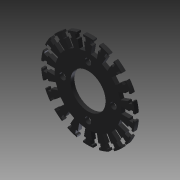
# Autodesk Inventor part: Plate 1
Saved by Autodesk Inventor 2015 (Build 190159000, 159)
## iProperties
Created: 2016-10-18
Part Number: Plate 1
Material: Generic
Document SubType Name: Modeling
Designer: James Yelland
Density: 1 g/cm^3
Appearance: Default
Author: James Yelland
Autodesk Inventor part; units mm, degrees
ref_plane "YZ Plane" through (0, 0, 0) normal (1, 0, 0) x (0, 1, 0)
ref_plane "XZ Plane" through (0, 0, 0) normal (0, 1, 0) x (-1, 0, 0)
ref_plane "XY Plane" through (0, 0, 0) normal (0, 0, 1) x (1, 0, 0)
sketch "Sketch1" plane through (0, 0, 0) normal (0, 1, 0) x (-1, 0, 0)
  circle A0 centre (0, 0) radius 24
  dimension "d0" = 48
  constraints: 1 centre point, 1 coincident
  measures "d0" diameter of A0
extrude "Extrusion1" add sketch "Sketch1" along normal blind 2
sketch "Sketch2" plane through (0, 2, 0) normal (0, 1, 0) x (1, 0, 0)
  line L0 (-24, 0) -> (-24, 1.6)
  line L1 (-24, 0) -> (-22.4, 0) construction
  line L2 (-17, 0.8) -> (-17, -0.8)
  line L3 (-24, -1.6) -> (-24, 1.6)
  line L4 (-24, 1.6) -> (-23, 1.6)
  line L5 (-23, 1.6) -> (-23, 2.6)
  line L6 (-23, 2.6) -> (-21, 2.6)
  line L7 (-21, 2.6) -> (-21, 1.6)
  line L8 (-17, -1.6) -> (-17, -0.8)
  line L9 (-17, 0.8) -> (-17, 1.6)
  line L10 (-24, -1.6) -> (-23, -1.6)
  line L11 (-23, -1.6) -> (-23, -2.6)
  line L12 (-23, -2.6) -> (-21, -2.6)
  line L13 (-21, -2.6) -> (-21, -1.6)
  line L14 (-21, -1.6) -> (-17, -1.6)
  line L15 (-17, 1.6) -> (-21, 1.6)
  line L16 (-22.5526, -8.2085) -> (-23.0999, -6.705)
  line L17 (-22.5526, -8.2085) -> (-21.0491, -7.6613) construction
  line L18 (-16.2484, -5.0626) -> (-15.7012, -6.5661)
  line L19 (-22.0054, -9.712) -> (-23.0999, -6.705)
  line L20 (-23.0999, -6.705) -> (-22.1602, -6.363)
  line L21 (-22.1602, -6.363) -> (-22.5022, -5.4233)
  line L22 (-22.5022, -5.4233) -> (-20.6228, -4.7392)
  line L23 (-20.6228, -4.7392) -> (-20.2808, -5.6789)
  line L24 (-15.4275, -7.3179) -> (-15.7012, -6.5661)
  line L25 (-16.2484, -5.0626) -> (-16.522, -4.3108)
  line L26 (-22.0054, -9.712) -> (-21.0657, -9.37)
  line L27 (-21.0657, -9.37) -> (-20.7237, -10.3097)
  line L28 (-20.7237, -10.3097) -> (-18.8443, -9.6256)
  line L29 (-18.8443, -9.6256) -> (-19.1863, -8.6859)
  line L30 (-19.1863, -8.6859) -> (-15.4275, -7.3179)
  line L31 (-16.522, -4.3108) -> (-20.2808, -5.6789)
  line L32 (-18.3851, -15.4269) -> (-19.4135, -14.2012)
  line L33 (-18.3851, -15.4269) -> (-17.1594, -14.3984) construction
  line L34 (-13.537, -10.3146) -> (-12.5085, -11.5402)
  line L35 (-17.3566, -16.6526) -> (-19.4135, -14.2012)
  line L36 (-19.4135, -14.2012) -> (-18.6475, -13.5584)
  line L37 (-18.6475, -13.5584) -> (-19.2903, -12.7924)
  line L38 (-19.2903, -12.7924) -> (-17.7582, -11.5068)
  line L39 (-17.7582, -11.5068) -> (-17.1154, -12.2729)
  line L40 (-11.9943, -12.1531) -> (-12.5085, -11.5402)
  line L41 (-13.537, -10.3146) -> (-14.0512, -9.7017)
  line L42 (-17.3566, -16.6526) -> (-16.5906, -16.0098)
  line L43 (-16.5906, -16.0098) -> (-15.9478, -16.7758)
  line L44 (-15.9478, -16.7758) -> (-14.4157, -15.4903)
  line L45 (-14.4157, -15.4903) -> (-15.0585, -14.7242)
  line L46 (-15.0585, -14.7242) -> (-11.9943, -12.1531)
  line L47 (-14.0512, -9.7017) -> (-17.1154, -12.2729)
  line L48 (-12, -20.7846) -> (-13.3856, -19.9846)
  line L49 (-12, -20.7846) -> (-11.2, -19.399) construction
  line L50 (-9.1928, -14.3224) -> (-7.8072, -15.1224)
  line L51 (-10.6144, -21.5846) -> (-13.3856, -19.9846)
  line L52 (-13.3856, -19.9846) -> (-12.8856, -19.1186)
  line L53 (-12.8856, -19.1186) -> (-13.7517, -18.6186)
  line L54 (-13.7517, -18.6186) -> (-12.7517, -16.8865)
  line L55 (-12.7517, -16.8865) -> (-11.8856, -17.3865)
  line L56 (-7.1144, -15.5224) -> (-7.8072, -15.1224)
  line L57 (-9.1928, -14.3224) -> (-9.8856, -13.9224)
  line L58 (-10.6144, -21.5846) -> (-10.1144, -20.7186)
  line L59 (-10.1144, -20.7186) -> (-9.2483, -21.2186)
  line L60 (-9.2483, -21.2186) -> (-8.2483, -19.4865)
  line L61 (-8.2483, -19.4865) -> (-9.1144, -18.9865)
  line L62 (-9.1144, -18.9865) -> (-7.1144, -15.5224)
  line L63 (-9.8856, -13.9224) -> (-11.8856, -17.3865)
  line L64 (-4.1676, -23.6354) -> (-5.7432, -23.3575)
  line L65 (-4.1676, -23.6354) -> (-3.8897, -22.0597) construction
  line L66 (-3.7399, -16.6028) -> (-2.1642, -16.8807)
  line L67 (-2.5919, -23.9132) -> (-5.7432, -23.3575)
  line L68 (-5.7432, -23.3575) -> (-5.5696, -22.3727)
  line L69 (-5.5696, -22.3727) -> (-6.5544, -22.1991)
  line L70 (-6.5544, -22.1991) -> (-6.2071, -20.2295)
  line L71 (-6.2071, -20.2295) -> (-5.2223, -20.4031)
  line L72 (-1.3763, -17.0196) -> (-2.1642, -16.8807)
  line L73 (-3.7399, -16.6028) -> (-4.5277, -16.4639)
  line L74 (-2.5919, -23.9132) -> (-2.4182, -22.9284)
  line L75 (-2.4182, -22.9284) -> (-1.4334, -23.1021)
  line L76 (-1.4334, -23.1021) -> (-1.0861, -21.1324)
  line L77 (-1.0861, -21.1324) -> (-2.0709, -20.9588)
  line L78 (-2.0709, -20.9588) -> (-1.3763, -17.0196)
  line L79 (-4.5277, -16.4639) -> (-5.2223, -20.4031)
  line L80 (4.1676, -23.6354) -> (2.5919, -23.9132)
  line L81 (4.1676, -23.6354) -> (3.8897, -22.0597) construction
  line L82 (2.1642, -16.8807) -> (3.7399, -16.6028)
  line L83 (5.7432, -23.3575) -> (2.5919, -23.9132)
  line L84 (2.5919, -23.9132) -> (2.4182, -22.9284)
  line L85 (2.4182, -22.9284) -> (1.4334, -23.1021)
  line L86 (1.4334, -23.1021) -> (1.0861, -21.1324)
  line L87 (1.0861, -21.1324) -> (2.0709, -20.9588)
  line L88 (4.5277, -16.4639) -> (3.7399, -16.6028)
  line L89 (2.1642, -16.8807) -> (1.3763, -17.0196)
  line L90 (5.7432, -23.3575) -> (5.5696, -22.3727)
  line L91 (5.5696, -22.3727) -> (6.5544, -22.1991)
  line L92 (6.5544, -22.1991) -> (6.2071, -20.2295)
  line L93 (6.2071, -20.2295) -> (5.2223, -20.4031)
  line L94 (5.2223, -20.4031) -> (4.5277, -16.4639)
  line L95 (1.3763, -17.0196) -> (2.0709, -20.9588)
  line L96 (12, -20.7846) -> (10.6144, -21.5846)
  line L97 (12, -20.7846) -> (11.2, -19.399) construction
  line L98 (7.8072, -15.1224) -> (9.1928, -14.3224)
  line L99 (13.3856, -19.9846) -> (10.6144, -21.5846)
  line L100 (10.6144, -21.5846) -> (10.1144, -20.7186)
  line L101 (10.1144, -20.7186) -> (9.2483, -21.2186)
  line L102 (9.2483, -21.2186) -> (8.2483, -19.4865)
  line L103 (8.2483, -19.4865) -> (9.1144, -18.9865)
  line L104 (9.8856, -13.9224) -> (9.1928, -14.3224)
  line L105 (7.8072, -15.1224) -> (7.1144, -15.5224)
  line L106 (13.3856, -19.9846) -> (12.8856, -19.1186)
  line L107 (12.8856, -19.1186) -> (13.7517, -18.6186)
  line L108 (13.7517, -18.6186) -> (12.7517, -16.8865)
  line L109 (12.7517, -16.8865) -> (11.8856, -17.3865)
  line L110 (11.8856, -17.3865) -> (9.8856, -13.9224)
  line L111 (7.1144, -15.5224) -> (9.1144, -18.9865)
  line L112 (18.3851, -15.4269) -> (17.3566, -16.6526)
  line L113 (18.3851, -15.4269) -> (17.1594, -14.3984) construction
  line L114 (12.5085, -11.5402) -> (13.537, -10.3146)
  line L115 (19.4135, -14.2012) -> (17.3566, -16.6526)
  line L116 (17.3566, -16.6526) -> (16.5906, -16.0098)
  line L117 (16.5906, -16.0098) -> (15.9478, -16.7758)
  line L118 (15.9478, -16.7758) -> (14.4157, -15.4903)
  line L119 (14.4157, -15.4903) -> (15.0585, -14.7242)
  line L120 (14.0512, -9.7017) -> (13.537, -10.3146)
  line L121 (12.5085, -11.5402) -> (11.9943, -12.1531)
  line L122 (19.4135, -14.2012) -> (18.6475, -13.5584)
  line L123 (18.6475, -13.5584) -> (19.2903, -12.7924)
  line L124 (19.2903, -12.7924) -> (17.7582, -11.5068)
  line L125 (17.7582, -11.5068) -> (17.1154, -12.2729)
  line L126 (17.1154, -12.2729) -> (14.0512, -9.7017)
  line L127 (11.9943, -12.1531) -> (15.0585, -14.7242)
  line L128 (22.5526, -8.2085) -> (22.0054, -9.712)
  line L129 (22.5526, -8.2085) -> (21.0491, -7.6613) construction
  line L130 (15.7012, -6.5661) -> (16.2484, -5.0626)
  line L131 (23.0999, -6.705) -> (22.0054, -9.712)
  line L132 (22.0054, -9.712) -> (21.0657, -9.37)
  line L133 (21.0657, -9.37) -> (20.7237, -10.3097)
  line L134 (20.7237, -10.3097) -> (18.8443, -9.6256)
  line L135 (18.8443, -9.6256) -> (19.1863, -8.6859)
  line L136 (16.522, -4.3108) -> (16.2484, -5.0626)
  line L137 (15.7012, -6.5661) -> (15.4275, -7.3179)
  line L138 (23.0999, -6.705) -> (22.1602, -6.363)
  line L139 (22.1602, -6.363) -> (22.5022, -5.4233)
  line L140 (22.5022, -5.4233) -> (20.6228, -4.7392)
  line L141 (20.6228, -4.7392) -> (20.2808, -5.6789)
  line L142 (20.2808, -5.6789) -> (16.522, -4.3108)
  line L143 (15.4275, -7.3179) -> (19.1863, -8.6859)
  line L144 (24, 0) -> (24, -1.6)
  line L145 (24, 0) -> (22.4, 0) construction
  line L146 (17, -0.8) -> (17, 0.8)
  line L147 (24, 1.6) -> (24, -1.6)
  line L148 (24, -1.6) -> (23, -1.6)
  line L149 (23, -1.6) -> (23, -2.6)
  line L150 (23, -2.6) -> (21, -2.6)
  line L151 (21, -2.6) -> (21, -1.6)
  line L152 (17, 1.6) -> (17, 0.8)
  line L153 (17, -0.8) -> (17, -1.6)
  line L154 (24, 1.6) -> (23, 1.6)
  line L155 (23, 1.6) -> (23, 2.6)
  line L156 (23, 2.6) -> (21, 2.6)
  line L157 (21, 2.6) -> (21, 1.6)
  line L158 (21, 1.6) -> (17, 1.6)
  line L159 (17, -1.6) -> (21, -1.6)
  line L160 (22.5526, 8.2085) -> (23.0999, 6.705)
  line L161 (22.5526, 8.2085) -> (21.0491, 7.6613) construction
  line L162 (16.2484, 5.0626) -> (15.7012, 6.5661)
  line L163 (22.0054, 9.712) -> (23.0999, 6.705)
  line L164 (23.0999, 6.705) -> (22.1602, 6.363)
  line L165 (22.1602, 6.363) -> (22.5022, 5.4233)
  line L166 (22.5022, 5.4233) -> (20.6228, 4.7392)
  line L167 (20.6228, 4.7392) -> (20.2808, 5.6789)
  line L168 (15.4275, 7.3179) -> (15.7012, 6.5661)
  line L169 (16.2484, 5.0626) -> (16.522, 4.3108)
  line L170 (22.0054, 9.712) -> (21.0657, 9.37)
  line L171 (21.0657, 9.37) -> (20.7237, 10.3097)
  line L172 (20.7237, 10.3097) -> (18.8443, 9.6256)
  line L173 (18.8443, 9.6256) -> (19.1863, 8.6859)
  line L174 (19.1863, 8.6859) -> (15.4275, 7.3179)
  line L175 (16.522, 4.3108) -> (20.2808, 5.6789)
  line L176 (18.3851, 15.4269) -> (19.4135, 14.2012)
  line L177 (18.3851, 15.4269) -> (17.1594, 14.3984) construction
  line L178 (13.537, 10.3146) -> (12.5085, 11.5402)
  line L179 (17.3566, 16.6526) -> (19.4135, 14.2012)
  line L180 (19.4135, 14.2012) -> (18.6475, 13.5584)
  line L181 (18.6475, 13.5584) -> (19.2903, 12.7924)
  line L182 (19.2903, 12.7924) -> (17.7582, 11.5068)
  line L183 (17.7582, 11.5068) -> (17.1154, 12.2729)
  line L184 (11.9943, 12.1531) -> (12.5085, 11.5402)
  line L185 (13.537, 10.3146) -> (14.0512, 9.7017)
  line L186 (17.3566, 16.6526) -> (16.5906, 16.0098)
  line L187 (16.5906, 16.0098) -> (15.9478, 16.7758)
  line L188 (15.9478, 16.7758) -> (14.4157, 15.4903)
  line L189 (14.4157, 15.4903) -> (15.0585, 14.7242)
  line L190 (15.0585, 14.7242) -> (11.9943, 12.1531)
  line L191 (14.0512, 9.7017) -> (17.1154, 12.2729)
  line L192 (12, 20.7846) -> (13.3856, 19.9846)
  line L193 (12, 20.7846) -> (11.2, 19.399) construction
  line L194 (9.1928, 14.3224) -> (7.8072, 15.1224)
  line L195 (10.6144, 21.5846) -> (13.3856, 19.9846)
  line L196 (13.3856, 19.9846) -> (12.8856, 19.1186)
  line L197 (12.8856, 19.1186) -> (13.7517, 18.6186)
  line L198 (13.7517, 18.6186) -> (12.7517, 16.8865)
  line L199 (12.7517, 16.8865) -> (11.8856, 17.3865)
  line L200 (7.1144, 15.5224) -> (7.8072, 15.1224)
  line L201 (9.1928, 14.3224) -> (9.8856, 13.9224)
  line L202 (10.6144, 21.5846) -> (10.1144, 20.7186)
  line L203 (10.1144, 20.7186) -> (9.2483, 21.2186)
  line L204 (9.2483, 21.2186) -> (8.2483, 19.4865)
  line L205 (8.2483, 19.4865) -> (9.1144, 18.9865)
  line L206 (9.1144, 18.9865) -> (7.1144, 15.5224)
  line L207 (9.8856, 13.9224) -> (11.8856, 17.3865)
  line L208 (4.1676, 23.6354) -> (5.7432, 23.3575)
  line L209 (4.1676, 23.6354) -> (3.8897, 22.0597) construction
  line L210 (3.7399, 16.6028) -> (2.1642, 16.8807)
  line L211 (2.5919, 23.9132) -> (5.7432, 23.3575)
  line L212 (5.7432, 23.3575) -> (5.5696, 22.3727)
  line L213 (5.5696, 22.3727) -> (6.5544, 22.1991)
  line L214 (6.5544, 22.1991) -> (6.2071, 20.2295)
  line L215 (6.2071, 20.2295) -> (5.2223, 20.4031)
  line L216 (1.3763, 17.0196) -> (2.1642, 16.8807)
  line L217 (3.7399, 16.6028) -> (4.5277, 16.4639)
  line L218 (2.5919, 23.9132) -> (2.4182, 22.9284)
  line L219 (2.4182, 22.9284) -> (1.4334, 23.1021)
  line L220 (1.4334, 23.1021) -> (1.0861, 21.1324)
  line L221 (1.0861, 21.1324) -> (2.0709, 20.9588)
  line L222 (2.0709, 20.9588) -> (1.3763, 17.0196)
  line L223 (4.5277, 16.4639) -> (5.2223, 20.4031)
  line L224 (-4.1676, 23.6354) -> (-2.5919, 23.9132)
  line L225 (-4.1676, 23.6354) -> (-3.8897, 22.0597) construction
  line L226 (-2.1642, 16.8807) -> (-3.7399, 16.6028)
  line L227 (-5.7432, 23.3575) -> (-2.5919, 23.9132)
  line L228 (-2.5919, 23.9132) -> (-2.4182, 22.9284)
  line L229 (-2.4182, 22.9284) -> (-1.4334, 23.1021)
  line L230 (-1.4334, 23.1021) -> (-1.0861, 21.1324)
  line L231 (-1.0861, 21.1324) -> (-2.0709, 20.9588)
  line L232 (-4.5277, 16.4639) -> (-3.7399, 16.6028)
  line L233 (-2.1642, 16.8807) -> (-1.3763, 17.0196)
  line L234 (-5.7432, 23.3575) -> (-5.5696, 22.3727)
  line L235 (-5.5696, 22.3727) -> (-6.5544, 22.1991)
  line L236 (-6.5544, 22.1991) -> (-6.2071, 20.2295)
  line L237 (-6.2071, 20.2295) -> (-5.2223, 20.4031)
  line L238 (-5.2223, 20.4031) -> (-4.5277, 16.4639)
  line L239 (-1.3763, 17.0196) -> (-2.0709, 20.9588)
  line L240 (-12, 20.7846) -> (-10.6144, 21.5846)
  line L241 (-12, 20.7846) -> (-11.2, 19.399) construction
  line L242 (-7.8072, 15.1224) -> (-9.1928, 14.3224)
  line L243 (-13.3856, 19.9846) -> (-10.6144, 21.5846)
  line L244 (-10.6144, 21.5846) -> (-10.1144, 20.7186)
  line L245 (-10.1144, 20.7186) -> (-9.2483, 21.2186)
  line L246 (-9.2483, 21.2186) -> (-8.2483, 19.4865)
  line L247 (-8.2483, 19.4865) -> (-9.1144, 18.9865)
  line L248 (-9.8856, 13.9224) -> (-9.1928, 14.3224)
  line L249 (-7.8072, 15.1224) -> (-7.1144, 15.5224)
  line L250 (-13.3856, 19.9846) -> (-12.8856, 19.1186)
  line L251 (-12.8856, 19.1186) -> (-13.7517, 18.6186)
  line L252 (-13.7517, 18.6186) -> (-12.7517, 16.8865)
  line L253 (-12.7517, 16.8865) -> (-11.8856, 17.3865)
  line L254 (-11.8856, 17.3865) -> (-9.8856, 13.9224)
  line L255 (-7.1144, 15.5224) -> (-9.1144, 18.9865)
  line L256 (-18.3851, 15.4269) -> (-17.3566, 16.6526)
  line L257 (-18.3851, 15.4269) -> (-17.1594, 14.3984) construction
  line L258 (-12.5085, 11.5402) -> (-13.537, 10.3146)
  line L259 (-19.4135, 14.2012) -> (-17.3566, 16.6526)
  line L260 (-17.3566, 16.6526) -> (-16.5906, 16.0098)
  line L261 (-16.5906, 16.0098) -> (-15.9478, 16.7758)
  line L262 (-15.9478, 16.7758) -> (-14.4157, 15.4903)
  line L263 (-14.4157, 15.4903) -> (-15.0585, 14.7242)
  line L264 (-14.0512, 9.7017) -> (-13.537, 10.3146)
  line L265 (-12.5085, 11.5402) -> (-11.9943, 12.1531)
  line L266 (-19.4135, 14.2012) -> (-18.6475, 13.5584)
  line L267 (-18.6475, 13.5584) -> (-19.2903, 12.7924)
  line L268 (-19.2903, 12.7924) -> (-17.7582, 11.5068)
  line L269 (-17.7582, 11.5068) -> (-17.1154, 12.2729)
  line L270 (-17.1154, 12.2729) -> (-14.0512, 9.7017)
  line L271 (-11.9943, 12.1531) -> (-15.0585, 14.7242)
  line L272 (-22.5526, 8.2085) -> (-22.0054, 9.712)
  line L273 (-22.5526, 8.2085) -> (-21.0491, 7.6613) construction
  line L274 (-15.7012, 6.5661) -> (-16.2484, 5.0626)
  line L275 (-23.0999, 6.705) -> (-22.0054, 9.712)
  line L276 (-22.0054, 9.712) -> (-21.0657, 9.37)
  line L277 (-21.0657, 9.37) -> (-20.7237, 10.3097)
  line L278 (-20.7237, 10.3097) -> (-18.8443, 9.6256)
  line L279 (-18.8443, 9.6256) -> (-19.1863, 8.6859)
  line L280 (-16.522, 4.3108) -> (-16.2484, 5.0626)
  line L281 (-15.7012, 6.5661) -> (-15.4275, 7.3179)
  line L282 (-23.0999, 6.705) -> (-22.1602, 6.363)
  line L283 (-22.1602, 6.363) -> (-22.5022, 5.4233)
  line L284 (-22.5022, 5.4233) -> (-20.6228, 4.7392)
  line L285 (-20.6228, 4.7392) -> (-20.2808, 5.6789)
  line L286 (-20.2808, 5.6789) -> (-16.522, 4.3108)
  line L287 (-15.4275, 7.3179) -> (-19.1863, 8.6859)
  point P0 (0, 0)
  dimension "d13" = 360
  dimension "d3" = 1.6
  dimension "d4" = 90
  dimension "d32" = 1
  dimension "d33" = 1
  dimension "d34" = 2
  dimension "d36" = 1
  dimension "d37" = 1
  dimension "d38" = 2
  dimension "d39" = 90
  dimension "d42" = 360
  constraints: 576 end point, 36 point on line, 4 perpendicular, 2 equal length, 1 horizontal, 1 vertical, 577 other
  measures "d3" distance of L0.start L0.end
  measures "d4" angle of L1 L0
  measures "d32" distance of L0.end L4.end
  measures "d33" distance of L4.end L5.end
  measures "d34" distance of L5.end L6.end
  measures "d36" distance of L3.start L10.end
  measures "d37" distance of L10.end L11.end
  measures "d38" distance of L11.end L12.end
  measures "d39" angle of L12 L11
extrude "Extrusion2" cut sketch "Sketch2" against normal blind 2
sketch "Sketch3" plane through (0, 2, 0) normal (0, 1, 0) x (1, 0, 0)
  circle A0 centre (-13, 0) radius 1.6
  circle A1 centre (0, -13) radius 1.6
  circle A2 centre (13, 0) radius 1.6
  circle A3 centre (0, 13) radius 1.6
  circle A4 centre (0, 0) radius 9
  dimension "d29" = 360
  dimension "d18" = 3.2
  dimension "d21" = 360
  dimension "d31" = 18
  constraints: 5 centre point, 1 coincident, 10 other
  measures "d18" diameter of A0
  measures "d31" diameter of A4
extrude "Extrusion3" cut sketch "Sketch3" against normal blind 2
body "Solid1"
